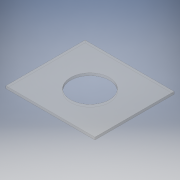
# Autodesk Inventor part: LexanBasePlate
Saved by Autodesk Inventor 2016 SP1 (Build 200210100, 210)
## iProperties
Created: 2015-11-03
Part Number: LexanBasePlate
Material: Polycarbonate, Clear
Document SubType Name: Modeling
Designer: steele
Mass: 353.961 g
Surface Area: 983.869 cm^2
Volume: 294.967 cm^3
Density: 1.2 g/cm^3
Appearance: Polycarbonate - Clear
Author: steele
Autodesk Inventor part; units mm, degrees
ref_plane "YZ Plane" through (0, 0, 0) normal (1, 0, 0) x (0, 1, 0)
ref_plane "XZ Plane" through (0, 0, 0) normal (0, 1, 0) x (-1, 0, 0)
ref_plane "XY Plane" through (0, 0, 0) normal (0, 0, 1) x (1, 0, 0)
sketch "Sketch2" plane through (0, 0, 0) normal (0, 1, 0) x (-1, 0, 0)
  line L0 (-114.3, 101.6) -> (-114.3, -101.6)
  line L1 (-114.3, -101.6) -> (114.3, -101.6)
  line L2 (114.3, -101.6) -> (114.3, 101.6)
  line L3 (114.3, 101.6) -> (-114.3, 101.6)
  line L4 (-114.3, 101.6) -> (114.3, -101.6) construction
  line L5 (-114.3, -101.6) -> (114.3, 101.6) construction
  point P0 (0, 0)
  dimension "d1" = 203.2
  dimension "d2" = 228.6
  constraints: 12 end point, 2 midpoint, 2 parallel, 1 perpendicular, 1 vertical
  measures "d1" distance of L0.start L0.end
  measures "d2" distance of L2.end L0.start
extrude "Extrusion1" add sketch "Sketch2" against normal blind 6.35
sketch "Sketch3" plane through (0, 0, 0) normal (0, 1, 0) x (1, 0, 0)
  circle A0 centre (0, 0) radius 49.7417
  dimension "d5" = 99.4833
  constraints: 1 centre point, 1 coincident
  measures "d5" diameter of A0
extrude "Extrusion2" cut sketch "Sketch3" against normal through all
equation "\"ringInnerDiam\" = 105.83333"
body "Solid1"
